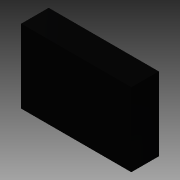
# Autodesk Inventor part: LTC2942
Saved by Autodesk Inventor 2013 (Build 170138000, 138)
## iProperties
Created: 2015-07-08
Part Number: LTC2942
Material: Ogólny
Document SubType Name: Modeling
Designer: terg
Density: 1 g/cm^3
Author: terg
Autodesk Inventor part; units mm, degrees
ref_plane "YZ Plane" through (0, 0, 0) normal (1, 0, 0) x (0, 1, 0)
ref_plane "XZ Plane" through (0, 0, 0) normal (0, 1, 0) x (-1, 0, 0)
ref_plane "XY Plane" through (0, 0, 0) normal (0, 0, 1) x (1, 0, 0)
sketch "Szkic1" plane through (0, 0, 0) normal (0, 1, 0) x (-1, 0, 0)
  line L0 (0, 0) -> (3, 0)
  line L1 (3, 0) -> (3, 2)
  line L2 (3, 2) -> (0, 2)
  line L3 (0, 2) -> (0, 0)
  dimension "d0" = 3
  dimension "d1" = 2
  constraints: 8 end point, 2 parallel, 1 horizontal, 1 perpendicular
  measures "d0" distance of L2.end L1.end
  measures "d1" distance of L1.end L0.end
extrude "Wyciągnięcie proste1" add sketch "Szkic1" along normal blind 0.75
sketch "Szkic2" plane through (0, 0.75, 0) normal (0, 1, 0) x (1, 0, 0)
  line L0 (0, 0) -> (-3, 0) projected
  line L1 (-3, 0) -> (-3, -2) projected
  line L2 (-3, -2) -> (0, -2) projected
  line L3 (-2.8, -0.15) -> (-2.65, -0.15)
  line L4 (-2.65, -0.15) -> (-2.65, -0.85)
  line L5 (-2.65, -0.85) -> (-2.8, -0.85)
  line L6 (-2.8, -0.85) -> (-2.8, -0.15)
  dimension "d4" = 0.15
  dimension "d5" = 0.2
  dimension "d6" = 0.7
  dimension "d11" = 1.15
  dimension "d12" = 0.15
  constraints: 8 end point, 2 parallel, 1 horizontal, 1 perpendicular
  measures "d4" distance of L4.end L5.end
  measures "d5" distance between parallel lines of L1 L6
  measures "d6" distance of L3.end L4.end
  measures "d11" distance between parallel lines of L2 L5
  measures "d12" distance between parallel lines of L0 L3
extrude "Wyciągnięcie proste2" cut sketch "Szkic2" against normal blind 0.1
